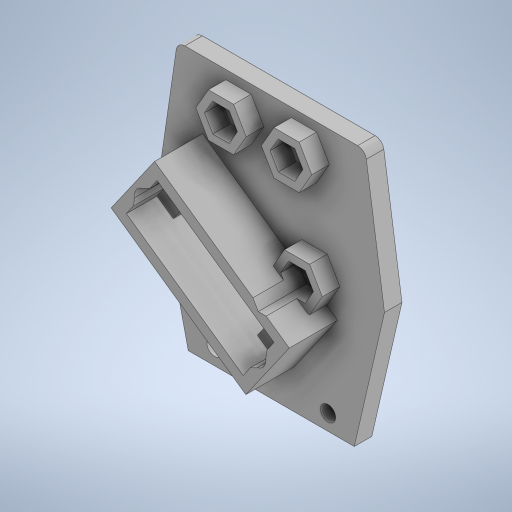
# Autodesk Inventor part: head
Saved by Autodesk Inventor 2023 (Build 270158000, 158)
## iProperties
Created: 2024-07-18
Part Number: head
Material: Generic
Document SubType Name: Modeling
Designer: Swoby
Density: 1 g/cm^3
Appearance: Default
Author: Swoby
Autodesk Inventor part; units mm, degrees
ref_plane "YZ Plane" through (0, 0, 0) normal (1, 0, 0) x (0, 1, 0)
ref_plane "XZ Plane" through (0, 0, 0) normal (0, 1, 0) x (-1, 0, 0)
ref_plane "XY Plane" through (0, 0, 0) normal (0, 0, 1) x (1, 0, 0)
sketch "Sketch1" plane through (0, 0, 0) normal (0, 0, 1) x (1, 0, 0)
  circle A0 centre (-7.5, 23) radius 2
  circle A1 centre (-9.9, 0) radius 2
  line L0 (0, 30) -> (-21.5, 30)
  line L1 (-21.5, 30) -> (-25.9, 0)
  line L2 (-25.9, 0) -> (-19, -30)
  line L3 (-19, -30) -> (0, -30)
  line L4 (0, -30) -> (0, 30) construction
  line L5 (-9.9, 0) -> (0, 0)
  line L6 (0, 30) -> (21.5, 30)
  line L7 (21.5, 30) -> (25.9, 0)
  line L8 (25.9, 0) -> (19, -30)
  line L9 (19, -30) -> (0, -30)
  circle A2 centre (7.5, 23) radius 2
  circle A3 centre (9.9, 0) radius 2
  dimension "d0" = 4
  dimension "d1" = 4
  dimension "d3" = 14
  dimension "d6" = 16
  dimension "d7" = 7
  dimension "d8" = 19
  dimension "d9" = 30
  dimension "d10" = 30
  dimension "d11" = 19
  dimension "d12" = 21.5
  dimension "d13" = 4
  dimension "d14" = 7
  dimension "d15" = 7.5
  dimension "d16" = 30
  dimension "d17" = 30
  dimension "d18" = 4
  dimension "d20" = 16
  dimension "d47" = 9.9
  dimension "d79" = 9.9
  dimension "d98" = 7.5
  constraints: 20 end point, 4 centre point, 2 collinear, 2 horizontal, 2 midpoint, 2 point on line, 1 coincident, 1 parallel, 1 perpendicular
  measures "d0" diameter of A0
  measures "d1" diameter of A1
  measures "d3" horizontal distance of A0.centre L0.end
  measures "d6" distance of L1.end A1.centre
  measures "d7" distance from line of L0 A0.centre
  measures "d8" distance of L2.end L3.end
  measures "d9" vertical distance of L1.end L0.end
  measures "d10" vertical distance of L1.end L2.end
  measures "d11" distance of L8.end L3.end
  measures "d12" distance of L0.start L6.end
  measures "d13" diameter of A2
  measures "d14" distance from line of L6 A2.centre
  measures "d15" horizontal distance of L0.start A2.centre
  measures "d16" vertical distance of L6.end L7.end
  measures "d17" vertical distance of L7.end L8.end
  measures "d18" diameter of A3
  measures "d20" distance of L7.end A3.centre
  measures "d47" distance of A3.centre L5.end
  measures "d79" distance of L5.end A1.centre
  measures "d98" distance from line of A0.centre L4
extrude "Extrusion1" add sketch "Sketch1" along normal blind 4
fillet "Fillet1" radius 2 2 edges at (-21.5, 30, 2) (21.5, 30, 2)
ref_plane "Work Plane1" through (0, 176.5909, 4) normal (1, 0, 0) x (0, 0, -1)
sketch "Sketch2" plane through (0, 0, 4) normal (0, 0, 1) x (1, 0, 0)
  circle A0 centre (-9.9, 0) radius 2 projected
  line L0 (-15.7104, 14.6282) -> (15.1061, -6.9498)
  line L1 (15.1061, -6.9498) -> (5.1832, -21.1211)
  line L2 (5.1832, -21.1211) -> (-25.6333, 0.4569)
  line L3 (-25.6333, 0.4569) -> (-15.7104, 14.6282)
  line L4 (-20.6718, 7.5425) -> (10.1447, -14.0354) construction
  line L5 (-15.0965, 11.1464) -> (11.6243, -7.5637)
  line L6 (11.6243, -7.5637) -> (4.5693, -17.6393)
  line L7 (4.5693, -17.6393) -> (-22.1515, 1.0708)
  line L8 (-22.1515, 1.0708) -> (-15.0965, 11.1464)
  line L9 (-15.0965, 11.1464) -> (-11.3693, 8.5366)
  line L10 (-11.3693, 8.5366) -> (-18.4243, -1.539)
  line L11 (-18.4243, -1.539) -> (-22.1515, 1.0708)
  line L12 (-22.1515, 1.0708) -> (-15.0965, 11.1464)
  line L13 (4.5693, -17.6393) -> (0.8421, -15.0295)
  line L14 (7.8971, -4.9539) -> (11.6243, -7.5637)
  line L15 (11.6243, -7.5637) -> (4.5693, -17.6393)
  line L16 (0, 42) -> (0, -42) projected
  line L17 (0.8421, -15.0295) -> (7.8971, -4.9539)
  dimension "d34" = 37.62
  dimension "d35" = 17.3
  dimension "d36" = 2.5
  dimension "d37" = 2.5
  dimension "d38" = 2.5
  dimension "d40" = 2.5
  dimension "d42" = 4.55
  dimension "d44" = 55
  dimension "d45" = 6.15
  dimension "d46" = 4.55
  dimension "d78" = 6.1
  constraints: 34 end point, 7 parallel, 4 perpendicular, 4 point on line, 2 midpoint
  measures "d34" distance of L0.start L0.end
  measures "d35" distance of L2.end L0.start
  measures "d36" distance between parallel lines of L5 L0
  measures "d37" distance between parallel lines of L3 L8
  measures "d38" distance between parallel lines of L1 L6
  measures "d40" distance between parallel lines of L2 L7
  measures "d42" distance of L10.end L11.end
  measures "d44" angle of L16 L0
  measures "d45" distance from line of L5 A0.centre
  measures "d46" distance between parallel lines of L15 L17
  measures "d78" distance from line of A0.centre L10
extrude "Extrusion2" add sketch "Sketch2" along normal blind 4 contours L10 L7 L8 L5 | L5 L6 L7 L17
extrude "Extrusion3" add sketch "Sketch2" along normal blind 11 contours L0 L16 L5 L8 L7 L2 L3 | L0 L1 L2 L16 L7 L6 L5
sketch "Sketch3" plane through (0, 0, 15) normal (0, 0, 1) x (1, 0, 0)
  line L0 (-15.7104, 14.6282) -> (-25.6333, 0.4569) projected
  line L1 (-25.6333, 0.4569) -> (5.1832, -21.1211) projected
  line L2 (5.1832, -21.1211) -> (15.1061, -6.9498) projected
  line L3 (15.1061, -6.9498) -> (-15.7104, 14.6282) projected
  line L4 (-15.0965, 11.1464) -> (11.6243, -7.5637) projected
  line L5 (11.6243, -7.5637) -> (4.5693, -17.6393) projected
  line L6 (4.5693, -17.6393) -> (-22.1515, 1.0708) projected
  line L7 (-22.1515, 1.0708) -> (-15.0965, 11.1464) projected
  line L8 (-18.624, 6.1086) -> (8.0968, -12.6015) construction
  circle A0 centre (-16.5269, 4.6402) radius 0.95
  circle A1 centre (5.9997, -11.1331) radius 0.95
  line L9 (-18.4243, -1.539) -> (-11.3693, 8.5366) projected
  line L10 (7.8971, -4.9539) -> (0.8421, -15.0295) projected
  arc A2 (-15.8617, 3.9621) -> (-17.3097, 7.9855) centre (-17.8048, 5.535) ccw construction
  arc A3 (6.7825, -14.4784) -> (9.411, -10.7246) centre (7.2776, -12.0279) ccw
  arc A4 (-19.9382, 4.2317) -> (-15.8617, 3.9621) centre (-17.8048, 5.535) ccw construction
  arc A5 (-17.3097, 7.9855) -> (-19.9382, 4.2317) centre (-17.8048, 5.535) ccw
  arc A6 (5.1349, -10.7399) -> (6.7825, -14.4784) centre (7.2776, -12.0279) ccw construction
  arc A7 (9.411, -10.7246) -> (5.1349, -10.7399) centre (7.2776, -12.0279) ccw construction
  point P0 (0, 0)
  dimension "d52" = 1.9
  dimension "d53" = 1.9
  dimension "d54" = 1.99
  dimension "d55" = 1.99
  dimension "d56" = 5
  dimension "d57" = 3.5
  dimension "d58" = 5
  dimension "d59" = 3.5
  constraints: 12 point on circle, 8 point on line, 6 centre point, 2 end point, 2 midpoint, 6 other
  measures "d54" distance from line of L9 point (-16.527, 4.64)
  measures "d55" distance from line of L10 point (6, -11.133)
  measures "d56" diameter of A2
  measures "d57" distance from line of A2.centre L0
  measures "d58" diameter of A3
  measures "d59" distance from line of L2 A3.centre
extrude "Extrusion4" cut sketch "Sketch3" against normal up to surface (7 mm away) contours L7 A5 | A3 L5
chamfer "Chamfer1" distance 1 angle 45 4 edges at (-17.3097, 7.9855, 11.5) (-19.9382, 4.2317, 11.5) (6.7825, -14.4784, 11.5) (9.411, -10.7246, 11.5)
extrude "Extrusion5" cut sketch "Sketch3" against normal blind 14 contours A0 | A1
sketch "Sketch4" plane through (0, 0, 4) normal (0, 0, 1) x (1, 0, 0)
  circle A0 centre (-9.9, 0) radius 2 projected
  line L0 (-18.4243, -1.539) -> (-11.3693, 8.5366) projected
  line L1 (-18.4243, -1.539) -> (0.8421, -15.0295) projected
  line L2 (0.8421, -15.0295) -> (7.8971, -4.9539) projected
  line L3 (7.8971, -4.9539) -> (-11.3693, 8.5366) projected
  line L4 (-11.3693, 8.5366) -> (-18.4243, -1.539) projected
  circle A1 centre (-9.9, 0) radius 2 projected
  arc A2 (-7.2134, -5.6984) -> (-4.0762, 2.4029) centre (-9.9, 0) ccw construction
  arc A3 (-5.241, -6.5026) -> (-2.1961, -2.154) centre (-5.108, -3.3554) ccw
  line L5 (-4.0762, 2.4029) -> (-2.1961, -2.154)
  line L6 (-10.1661, -6.2944) -> (-5.241, -6.5026)
  line L7 (-14.8968, 3.4988) -> (4.3696, -9.9917) construction
  arc A4 (-10.1661, -6.2944) -> (-7.2134, -5.6984) centre (-9.9, 0) ccw construction
  arc A5 (-7.2134, -5.6984) -> (-5.241, -6.5026) centre (-5.108, -3.3554) ccw construction
  arc A6 (-4.0762, 2.4029) -> (-10.1661, -6.2944) centre (-9.9, 0) ccw
  arc A7 (-2.1961, -2.154) -> (-7.2134, -5.6984) centre (-5.108, -3.3554) ccw construction
  point P0 (0, 0)
  point P1 (-5.2531, 4.254)
  point P2 (-7.4919, 5.8216)
  point P3 (-13.9936, 4.7888)
  point P4 (-15.8001, 2.2088)
  point P5 (-14.5469, -4.254)
  point P6 (-12.3081, -5.8216)
  dimension "d73" = 12.6
  dimension "d74" = 6.3
  dimension "d75" = 5.85
  constraints: 12 point on circle, 8 tangent, 6 centre point, 6 end point, 2 midpoint, 1 coincident, 1 point on line
  measures "d73" diameter of A2
  measures "d74" diameter of A3
  measures "d75" distance of A3.centre A0.centre
extrude "Extrusion6" cut sketch "Sketch4" against normal through all contours L0 A6 L3 L5 A3 L6 L1
sketch "Sketch5" plane through (0, 0, 4) normal (0, 0, 1) x (1, 0, 0)
  circle A0 centre (-7.5, 23) radius 2 projected
  circle A1 centre (7.5, 23) radius 2 projected
  circle A2 centre (9.9, 0) radius 2 projected
  line L0 (-5.6236, 26.25) -> (-3.7472, 23)
  line L1 (-3.7472, 23) -> (-5.6236, 19.75)
  line L2 (-5.6236, 19.75) -> (-9.3764, 19.75)
  line L3 (-9.3764, 19.75) -> (-11.2528, 23)
  line L4 (-11.2528, 23) -> (-9.3764, 26.25)
  line L5 (-9.3764, 26.25) -> (-5.6236, 26.25)
  line L6 (9.3764, 26.25) -> (11.2528, 23)
  line L7 (11.2528, 23) -> (9.3764, 19.75)
  line L8 (9.3764, 19.75) -> (5.6236, 19.75)
  line L9 (5.6236, 19.75) -> (3.7472, 23)
  line L10 (3.7472, 23) -> (5.6236, 26.25)
  line L11 (5.6236, 26.25) -> (9.3764, 26.25)
  line L12 (11.7764, 3.25) -> (13.6528, 0)
  line L13 (13.6528, 0) -> (11.7764, -3.25)
  line L14 (11.7764, -3.25) -> (8.0236, -3.25)
  line L15 (8.0236, -3.25) -> (6.1472, 0)
  line L16 (6.1472, 0) -> (8.0236, 3.25)
  line L17 (8.0236, 3.25) -> (11.7764, 3.25)
  line L18 (-4.6132, 28) -> (-1.7265, 23)
  line L19 (-1.7265, 23) -> (-4.6132, 18)
  line L20 (-4.6132, 18) -> (-10.3868, 18)
  line L21 (-10.3868, 18) -> (-13.2735, 23)
  line L22 (-13.2735, 23) -> (-10.3868, 28)
  line L23 (-10.3868, 28) -> (-4.6132, 28)
  line L24 (4.6132, 18) -> (10.3868, 18)
  line L25 (10.3868, 18) -> (13.2735, 23)
  line L26 (13.2735, 23) -> (10.3868, 28)
  line L27 (10.3868, 28) -> (4.6132, 28)
  line L28 (4.6132, 28) -> (1.7265, 23)
  line L29 (1.7265, 23) -> (4.6132, 18)
  line L30 (12.7868, 5) -> (15.6735, 0)
  line L31 (15.6735, 0) -> (12.7868, -5)
  line L32 (12.7868, -5) -> (7.9629, -5)
  line L33 (7.0132, -5) -> (6.3688, -3.8838) construction
  line L34 (4.1265, 0) -> (7.0132, 5)
  line L35 (7.0132, 5) -> (12.7868, 5)
  line L36 (-15.0965, 11.1464) -> (11.6243, -7.5637) projected
  line L37 (6.3688, -3.8838) -> (4.1265, 0)
  line L38 (7.9629, -5) -> (7.0132, -5) construction
  point P0 (0, 0)
  point P1 (9.9, 3.25)
  dimension "d80" = 6.5
  dimension "d81" = 6.5
  dimension "d82" = 6.5
  dimension "d85" = 10
  dimension "d86" = 10
  dimension "d87" = 10
  constraints: 76 end point, 3 coincident, 3 horizontal, 2 point on line, 1 midpoint, 51 other
  measures "d80" distance between parallel lines of L2 L5
  measures "d81" distance between parallel lines of L8 L11
  measures "d82" distance from line of L14 point (9.9, 3.25)
  measures "d85" distance between parallel lines of L20 L23
  measures "d86" distance between parallel lines of L27 L24
  measures "d87" distance between parallel lines of L32 L35
extrude "Extrusion7" cut sketch "Sketch5" along normal through all contours A2 | L12 L13 L14 L15 L16 L17
extrude "Extrusion8" add sketch "Sketch5" along normal blind 4 contours L18 L19 L20 L21 L22 L23 | L29 L28 L27 L26 L25 L24 | L30 L31 L32 L36 L37 L34 L35
sketch "Sketch6" plane through (0, 0, 0) normal (0, 0, -1) x (-1, 0, 0)
  circle A0 centre (-13, -26.4) radius 1.75
  circle A1 centre (13, -26.4) radius 1.75
  line L0 (19, -30) -> (-19, -30) projected
  point P0 (0, 0)
  dimension "d90" = 3.5
  dimension "d91" = 3.5
  dimension "d92" = 26
  dimension "d93" = 13
  dimension "d94" = 3.6
  dimension "d95" = 3.6
  constraints: 2 centre point
  measures "d90" diameter of A0
  measures "d91" diameter of A1
  measures "d92" distance of A1.centre A0.centre
  measures "d93" horizontal distance of point (0, 0) A0.centre
  measures "d94" distance from line of L0 A0.centre
  measures "d95" distance from line of L0 A1.centre
extrude "Extrusion9" cut sketch "Sketch6" against normal through all
equation "\"d1\" = d0"
equation "\"d11\" = d8"
equation "\"d13\" = d0"
equation "\"d14\" = d7"
equation "\"d18\" = d0"
equation "\"d47\" = d79"
equation "\"d81\" = d80"
equation "\"d82\" = d81"
equation "\"d86\" = d85"
equation "\"d87\" = d86"
equation "\"d95\" = d94"
body "Solid1"
